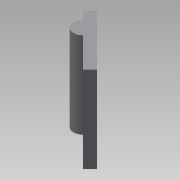
# Autodesk Inventor part: 17_Spiegelhalterung
Saved by Autodesk Inventor 2015 (Build 190159000, 159)
## iProperties
Created: 2016-03-16
Part Number: 17_Spiegelhalterung
Material: Generisch
Document SubType Name: Modeling
Designer: Bene
Density: 1 g/cm^3
Appearance: Vorgabe
Author: Bene
Autodesk Inventor part; units mm, degrees
ref_plane "YZ Plane" through (0, 0, 0) normal (1, 0, 0) x (0, 1, 0)
ref_plane "XZ Plane" through (0, 0, 0) normal (0, 1, 0) x (-1, 0, 0)
ref_plane "XY Plane" through (0, 0, 0) normal (0, 0, 1) x (1, 0, 0)
sketch "Skizze1" plane through (0, 0, 0) normal (0, 0, 1) x (1, 0, 0)
  circle A0 centre (13.0004, 19) radius 2.5 projected
  arc A1 (45.6946, 0) -> (10.6946, 35) centre (10.6946, 0) ccw projected
  line L0 (-4, 35) -> (10.6946, 35) projected
  line L1 (-4, 0) -> (-4, 35) projected
  line L2 (45.6946, 0) -> (-4, 0) projected
  line L3 (13.0004, -80.4986) -> (13.0004, 19) construction
  line L4 (13.0004, 19) -> (-57.6019, 19) construction
  line L5 (13.0004, 19) -> (40.4873, -8.4869) construction
  line L6 (13.0004, 19) -> (51.8727, 19) construction
  line L7 (32.0004, 0) -> (5.4793, 26.5211)
  line L8 (5.4793, 26.5211) -> (9.215, 30.2568)
  line L9 (9.215, 30.2568) -> (35.7361, 3.7357)
  line L10 (35.7361, 3.7357) -> (32.0004, 0)
  circle A2 centre (13.0004, 19) radius 4.9033
  line L11 (32.0004, 0) -> (35.7361, 3.7357)
  line L12 (35.7361, 3.7357) -> (44.223, -4.7511)
  line L13 (44.223, -4.7511) -> (40.4873, -8.4869)
  line L14 (40.4873, -8.4869) -> (32.0004, 0)
  point P0 (0, 0)
  dimension "d0" = 45
  constraints: 24 end point, 4 parallel, 4 perpendicular, 3 point on line, 1 centre point, 1 coincident, 1 equal length, 1 horizontal, 1 vertical
  measures "d0" angle of L5 L6
extrude "Extrusion1" add sketch "Skizze1" along normal blind 45 contours A0 L7 | A0 L7 A2 | L7 A0 | A0 L7 A2 | L7 L8 L9 L10 A2 | L10 L12 L2 | L2 L12 L13 L14
sketch "Skizze2" plane through (0, 0, 45) normal (0, 0, 1) x (1, 0, 0)
  circle A0 centre (13.0004, 19) radius 2.5 projected
  point P0 (0, 0)
extrude "Extrusion2" cut sketch "Skizze2" against normal through all
sketch "Skizze3" plane through (9.215, 30.2568, 0) normal (0.7071, 0.7071, 0) x (-0.7071, 0.7071, 0)
  point P0 (-14.8788, 0)
sketch "Skizze4" plane through (9.215, 30.2568, 0) normal (0.7071, 0.7071, 0) x (-0.7071, 0.7071, 0)
  line L0 (-49.5087, 0) -> (0, 0) projected
  line L1 (0, 0) -> (0, 45) projected
  line L2 (-49.5087, 45) -> (0, 45) projected
  line L3 (-49.5087, 0) -> (-49.5087, 45) projected
  line L4 (-3.2544, 2.717) -> (-46.2544, 2.717)
  line L5 (-46.2544, 2.717) -> (-46.2544, 40.717)
  line L6 (-46.2544, 40.717) -> (-3.2544, 40.717)
  line L7 (-3.2544, 40.717) -> (-3.2544, 2.717)
  line L8 (-3.2544, 2.717) -> (-46.2544, 40.717) construction
  line L9 (-46.2544, 2.717) -> (-3.2544, 40.717) construction
  point P0 (-14.8788, 0)
  point P1 (-24.7544, 21.717)
  dimension "d5" = 43
  dimension "d6" = 38
  constraints: 12 end point, 2 midpoint, 2 parallel, 1 horizontal, 1 perpendicular
  measures "d5" distance of L5.end L6.end
  measures "d6" distance of L4.end L5.end
extrude "Extrusion3" cut sketch "Skizze4" against normal blind 12 contours L4 L5 L6 L7
sketch "Skizze6" plane through (5.4793, 26.5211, 0) normal (-0.7071, 0.7071, 0) x (-0.7071, -0.7071, 0)
  line L0 (-5.2831, 0) -> (0, 0) projected
  line L1 (0, 0) -> (0, 45) projected
  line L2 (-5.2831, 45) -> (0, 45) projected
  line L3 (-5.2831, 0) -> (-5.2831, 45) projected
  line L4 (-4.1416, 1.5) -> (-1.1416, 1.5)
  line L5 (-1.1416, 1.5) -> (-1.1416, 43.5)
  line L6 (-1.1416, 43.5) -> (-4.1416, 43.5)
  line L7 (-4.1416, 43.5) -> (-4.1416, 1.5)
  line L8 (-4.1416, 1.5) -> (-1.1416, 43.5) construction
  line L9 (-1.1416, 1.5) -> (-4.1416, 43.5) construction
  point P0 (22.6277, 0)
  point P1 (-2.6416, 22.5)
  dimension "d11" = 3
  dimension "d12" = 42
  constraints: 12 end point, 2 midpoint, 2 parallel, 1 horizontal, 1 perpendicular
  measures "d11" distance of L6.end L5.end
  measures "d12" distance of L5.end L4.end
extrude "Extrusion5" cut sketch "Skizze6" against normal up to surface (46.2544 mm away) contours L7 L6 L5 L4
